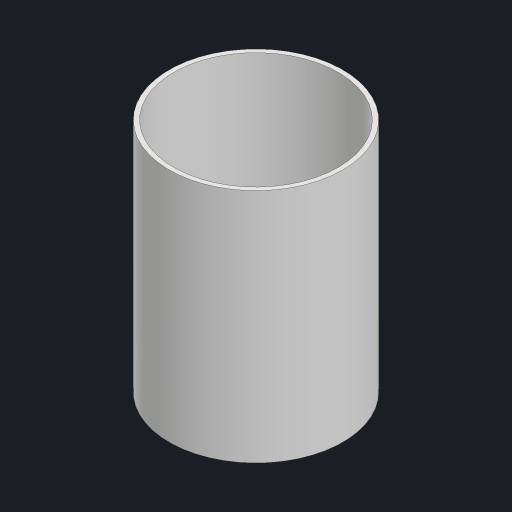
# Autodesk Inventor part: tulejka
Saved by Autodesk Inventor 2023 (Build 270158000, 158)
## iProperties
Created: 2024-06-19
Part Number: tulejka
Material: Generic
Document SubType Name: Modeling
Designer: szymo
Density: 1 g/cm^3
Appearance: Default
Author: szymo
Autodesk Inventor part; units mm, degrees
ref_plane "YZ Plane" through (0, 0, 0) normal (1, 0, 0) x (0, 1, 0)
ref_plane "XZ Plane" through (0, 0, 0) normal (0, 1, 0) x (-1, 0, 0)
ref_plane "XY Plane" through (0, 0, 0) normal (0, 0, 1) x (1, 0, 0)
ref_plane "Work Plane1" through (-16.584, 2, -16.584) normal (0, 1, 0) x (0.3814299, 0, 0.9243978)
sketch "Sketch1" plane through (0, 0, 0) normal (0, 1, 0) x (-1, 0, 0)
  circle A0 centre (0, 0) radius 22.5
  circle A1 centre (0, 0) radius 19.5
  circle A2 centre (0, 0) radius 12.7 projected
  circle A3 centre (0, 0) radius 6 projected
  circle A4 centre (8.8049, 3.6331) radius 1.63 projected
  circle A5 centre (7.5488, -5.8087) radius 1.63 projected
  circle A6 centre (-1.2561, -9.4418) radius 1.63 projected
  circle A7 centre (-8.8049, -3.6331) radius 1.63 projected
  circle A8 centre (-7.5488, 5.8087) radius 1.63 projected
  circle A9 centre (1.2561, 9.4418) radius 1.63 projected
  circle A10 centre (0, 0) radius 12.85
  dimension "d0" = 45
  dimension "d1" = 3
  dimension "d4" = 0.15
  constraints: 3 centre point, 2 coincident
  measures "d0" diameter of A0
  measures "d1" radial gap between concentric circles of A0 A1
  measures "d4" radial gap between concentric circles of A2 A10
extrude "Extrusion1" add sketch "Sketch1" along normal blind 2 contours A1
sketch "Sketch4" plane through (0, 2, 0) normal (0, 1, 0) x (1, 0, 0)
  circle A0 centre (0, 0) radius 22.5
  circle A1 centre (0, 0) radius 19.5
  circle A2 centre (0, 0) radius 18.5
  dimension "d13" = 45
  dimension "d14" = 3
  dimension "d15" = 1
  constraints: 3 centre point, 1 coincident
  measures "d13" diameter of A0
  measures "d14" radial gap between concentric circles of A0 A1
  measures "d15" radial gap between concentric circles of A1 A2
extrude "Extrusion4" add sketch "Sketch4" along normal blind 51 contours A1
fillet "Fillet2" radius 1 1 edges at (12.85, 0, 0)
body "Solid1"
